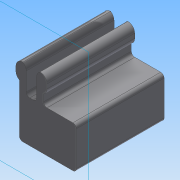
# Autodesk Inventor part: ledholder
Saved by Autodesk Inventor 2014 SP2 (Build 180246200, 246)
## iProperties
Created: 2014-07-18
Part Number: ledholder
Material: Generic
Document SubType Name: Modeling
Designer: dliu
Density: 1 g/cm^3
Appearance: Default
Author: dliu
Autodesk Inventor part; units mm, degrees
ref_plane "YZ Plane" through (0, 0, 0) normal (1, 0, 0) x (0, 1, 0)
ref_plane "XZ Plane" through (0, 0, 0) normal (0, 1, 0) x (-1, 0, 0)
ref_plane "XY Plane" through (0, 0, 0) normal (0, 0, 1) x (1, 0, 0)
sketch "Sketch1" plane through (0, 0, 0) normal (0, 1, 0) x (-1, 0, 0)
  line L0 (0, 0) -> (-16.5, 0)
  line L1 (-16.5, 0) -> (-16.5, -12)
  line L2 (-16.5, -12) -> (0, -12)
  line L3 (0, -12) -> (0, 0)
  line L4 (-5, 0) -> (-7, 0)
  line L5 (-7, 0) -> (-7, 8)
  line L6 (-7, 8) -> (-5, 8)
  line L7 (-5, 8) -> (-5, 0)
  line L8 (0, 0) -> (-2, 0)
  line L9 (-2, 0) -> (-2, 8)
  line L10 (-2, 8) -> (0, 8)
  line L11 (0, 8) -> (0, 0)
  line L12 (0, 8) -> (1, 8)
  line L13 (1, 8) -> (1, 3)
  line L14 (1, 3) -> (0, 3)
  line L15 (0, 3) -> (0, 8)
  line L16 (-7, 8) -> (-8, 8)
  line L17 (-8, 8) -> (-8, 3)
  line L18 (-8, 3) -> (-7, 3)
  line L19 (-7, 3) -> (-7, 8)
  dimension "d0" = 16.5
  dimension "d1" = 12
  dimension "d4" = 2
  dimension "d5" = 8
  dimension "d6" = 3
  dimension "d9" = 1
  dimension "d10" = 5
  constraints: 40 end point, 10 parallel, 5 horizontal, 5 perpendicular, 4 equal length, 1 point on line
  measures "d0" distance of L2.end L1.end
  measures "d1" distance of L1.end L0.end
  measures "d4" distance of L9.end L10.end
  measures "d5" distance of L8.end L9.end
  measures "d6" distance between parallel lines of L9 L7
  measures "d9" distance of L13.end L14.end
  measures "d10" distance of L12.end L13.end
extrude "Extrusion1" add sketch "Sketch1" along normal blind 25.4
fillet "Fillet1" radius 2 4 edges at (8, 12.7, 3) (8, 12.7, 8) (-1, 12.7, 3) (-1, 12.7, 8)
fillet "Fillet2" radius 1 3 edges at (16.5, 12.7, 0) (16.5, 12.7, -12) (0, 12.7, -12)
fillet "Fillet3" radius 1 3 edges at (5, 12.7, 0) (2, 12.7, 0) (7, 12.7, 0)
fillet "Fillet4" radius 2 2 edges at (5, 12.7, 8) (2, 12.7, 8)
body "Solid1"
